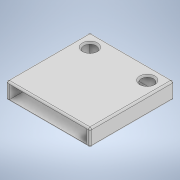
# Autodesk Inventor part: BaseBox
Saved by Autodesk Inventor 2022 (Build 260153000, 153)
## iProperties
Created: 2022-08-22
Part Number: BaseBox
Material: Generic
Document SubType Name: Modeling
Designer: sgioj
Density: 1 g/cm^3
Appearance: Default
Author: sgioj
Autodesk Inventor part; units mm, degrees
ref_plane "YZ Plane" through (0, 0, 0) normal (1, 0, 0) x (0, 1, 0)
ref_plane "XZ Plane" through (0, 0, 0) normal (0, 1, 0) x (-1, 0, 0)
ref_plane "XY Plane" through (0, 0, 0) normal (0, 0, 1) x (1, 0, 0)
sketch "Sketch1" plane through (0, 0, 0) normal (0, 0, 1) x (1, 0, 0)
  line L0 (-24, 5) -> (24, 5)
  line L1 (24, 5) -> (24, -5)
  line L2 (24, -5) -> (-24, -5)
  line L3 (-24, -5) -> (-24, 5)
  line L4 (-24, 5) -> (24, -5) construction
  line L5 (24, 5) -> (-24, -5) construction
  point P0 (0, 0)
  dimension "d0" = 48
  dimension "d1" = 10
  constraints: 12 end point, 2 midpoint, 2 parallel, 1 horizontal, 1 perpendicular
  measures "d0" distance of L1.end L2.end
  measures "d1" distance of L0.end L1.end
extrude "Extrusion1" add sketch "Sketch1" along normal blind 49
shell "Shell1" thickness 1 removed faces 1 at (8, -1.6667, 49)
sketch "Sketch2" plane through (-24, 5, 0) normal (0, 1, 0) x (1, 0, 0)
  line L0 (0, 0) -> (0, -49) projected
  line L1 (0, 0) -> (6.947, 0)
  line L2 (6.947, 0) -> (6.947, -6.947)
  line L3 (6.947, -6.947) -> (0, -6.947)
  line L4 (0, -6.947) -> (0, 0)
  line L5 (48, 0) -> (48, -49) projected
  line L6 (48, 0) -> (41.053, 0)
  line L7 (41.053, 0) -> (41.053, -6.947)
  line L8 (41.053, -6.947) -> (48, -6.947)
  line L9 (48, -6.947) -> (48, 0)
  point P0 (24, 0)
  dimension "d5" = 6.947
  dimension "d6" = 6.947
  dimension "d7" = 6.947
  dimension "d8" = 6.947
  constraints: 16 end point, 4 parallel, 2 coincident, 2 horizontal, 2 perpendicular
  measures "d5" distance of L2.end L3.end
  measures "d6" distance of L1.end L2.end
  measures "d7" distance of L8.end L7.end
  measures "d8" distance of L7.end L6.end
hole "Hole1" at (-17.053, 5, 6.947) at (17.053, 5, 6.947) direction (0, -1, 0) diameter 4.915 end through all countersink diameter 9 countersink angle 82 clearance for "Flat Head Machine Screw (82)" size "#8" standard "Ansi Unified Screw Threads"
move faces "Move1" translate (1, 0, 0) faces at (24, -1.6667, 32.6667)
move faces "Move2" translate (-1, 0, 0) faces at (-24, 1.6667, 32.6667)
move faces "Move3" translate (0, 0, -1) faces at (8.3333, -1.6667, 0)
fillet "Fillet1" radius 1 12 edges at (-25, 5, 24) (25, 5, 24) (0, 5, 49) (25, 0, 49) (0, -5, 49) (-25, 0, 49) (-25, -5, 24) (25, -5, 24) (25, 0, -1) (-25, 0, -1) (0, 5, -1) (0, -5, -1)
body "Solid1"
